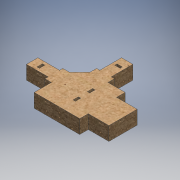
# Autodesk Inventor part: BearingStand
Saved by Autodesk Inventor 2016 (Build 200138000, 138)
## iProperties
Created: 2015-11-23
Part Number: BearingStand
Material: MDF Medium Density Fiberboard
Document SubType Name: Modeling
Designer: m2memari
Density: 0.8 g/cm^3
Appearance: Cardboard - Corrugated
BearingDiameter: 24.000 mm
WoodThickness: 6.390 mm
BearingWidth: 7.000 mm
BearingShaftDiameter: 8.000 mm
ZipTieWidth: 2.500 mm
ZipTieThickness: 1.100 mm
ZipTieClearance: 1.000 mm
ZipTieDistance: 10.000 mm
BearingShaftOffset: 1.574 mm
BearingHolderHeight: 23.674 mm
LatchHeight: 13.147 mm
BearingSiliconeWidth: 13.200 mm
Author: m2memari
Autodesk Inventor part; units mm, degrees
ref_plane "YZ Plane" through (0, 0, 0) normal (1, 0, 0) x (0, 1, 0)
ref_plane "XZ Plane" through (0, 0, 0) normal (0, 1, 0) x (-1, 0, 0)
ref_plane "XY Plane" through (0, 0, 0) normal (0, 0, 1) x (1, 0, 0)
sketch "Sketch1" plane through (0, 0, 0) normal (0, 0, 1) x (1, 0, 0)
  line L0 (-2.6473, 22.1) -> (2.6473, 22.1)
  line L1 (2.6473, 22.1) -> (2.6473, 12)
  line L2 (2.6473, 12) -> (4.1473, 12)
  line L3 (4.1473, 12) -> (4.1473, 9)
  line L4 (4.1473, 9) -> (12.1473, 9)
  line L5 (0, 22.1) -> (0, 0) construction
  line L6 (-2.6473, 22.1) -> (-2.6473, 12)
  line L7 (-2.6473, 12) -> (-4.1473, 12)
  line L8 (-1.25, 18.6) -> (1.25, 18.6)
  line L9 (1.25, 18.6) -> (1.25, 17.5)
  line L10 (1.25, 17.5) -> (-1.25, 17.5)
  line L11 (-1.25, 17.5) -> (-1.25, 18.6)
  line L12 (-5, -12.1473) -> (12.1473, -12.1473)
  line L13 (12.1473, 9) -> (12.1473, 5)
  line L14 (12.1473, 5) -> (21.7323, 5)
  line L15 (21.7323, -8.1473) -> (12.1473, -8.1473)
  line L16 (12.1473, -8.1473) -> (12.1473, -12.1473)
  line L17 (3.0473, 3) -> (4.1473, 3)
  line L18 (4.1473, 3) -> (4.1473, 0.5)
  line L19 (4.1473, 0.5) -> (3.0473, 0.5)
  line L20 (3.0473, 0.5) -> (3.0473, 3)
  line L21 (-4.1473, 12) -> (-19.8527, 12) construction
  line L22 (0, 0) -> (-12, 12) construction
  line L23 (-22.1, 2.6473) -> (-22.1, -2.6473)
  line L24 (-22.1, -2.6473) -> (-12, -2.6473)
  line L25 (-12, -2.6473) -> (-12, -4.1473)
  line L26 (-12, -4.1473) -> (-9, -4.1473)
  line L27 (-9, -4.1473) -> (-9, -12.1473)
  line L28 (-22.1, 2.6473) -> (-12, 2.6473)
  line L29 (-12, 2.6473) -> (-12, 4.1473)
  line L30 (-18.6, 1.25) -> (-18.6, -1.25)
  line L31 (-18.6, -1.25) -> (-17.5, -1.25)
  line L32 (-17.5, -1.25) -> (-17.5, 1.25)
  line L33 (-17.5, 1.25) -> (-18.6, 1.25)
  line L34 (-9, -12.1473) -> (-5, -12.1473)
  line L35 (-12, 12) -> (-12, -12.1473) construction
  line L36 (-4.1473, 12) -> (-4.1473, 9)
  line L37 (-9, 4.1473) -> (-12, 4.1473)
  line L38 (-4.1473, 9) -> (-9, 4.1473)
  line L39 (21.7323, 5) -> (21.7323, -8.1473)
  line L40 (21.7323, -1.5737) -> (3.3412, -1.5737) construction
  line L41 (3.0473, -6.1473) -> (4.1473, -6.1473)
  line L42 (4.1473, -6.1473) -> (4.1473, -3.6473)
  line L43 (4.1473, -3.6473) -> (3.0473, -3.6473)
  line L44 (3.0473, -3.6473) -> (3.0473, -6.1473)
  line L45 (-22.1, 0) -> (21.7323, 0) construction
  point P0 (0, 17.5)
  point P1 (3.0473, 1.75)
  point P2 (-17.5, 0)
  point P3 (4.1473, 1.75)
  point P4 (4.1473, 10.5)
  dimension "d4" = 1.5
  dimension "d5" = 3
  dimension "d26" = 10.1
  dimension "d27" = 5.2946
  dimension "d31" = 2.5
  dimension "d32" = 1.1
  dimension "d35" = 5.5
  dimension "d37" = 9.585
  dimension "d41" = 1.1
  dimension "d42" = 2.5
  dimension "d45" = 2
  dimension "d61" = 45
  dimension "d70" = 8
  dimension "d72" = 12
  dimension "BearingShaftOffset" = 1.5737
  dimension "BearingHolderHeight" = 23.6737
  dimension "LatchHeight" = 13.1473
  dimension "d95" = 24.1473
  constraints: 92 end point, 22 symmetric about line, 11 perpendicular, 7 midpoint, 6 horizontal, 5 parallel, 4 vertical, 3 vertical alignment, 2 collinear, 2 point on line
  measures "d4" distance of L1.end L2.end
  measures "d5" distance of L2.end L3.end
  measures "d26" distance of L0.end L1.end
  measures "d27" distance of L0.start L0.end
  measures "d31" distance of L8.start L8.end
  measures "d32" distance of L8.end L9.end
  measures "d35" distance between parallel lines of L7 L10
  measures "d37" distance of L13.end L14.end
  measures "d41" distance of L18.end L19.end
  measures "d42" distance of L17.end L18.end
  measures "d45" distance between parallel lines of L14 L17
  measures "d61" angle of L5 L22
  measures "d70" distance of L3.end L4.end
  measures "d72" distance between parallel lines of L35 L5
  measures "BearingShaftOffset" distance between parallel lines of L40 L45
  measures "BearingHolderHeight" distance between parallel lines of L40 L0
  measures "LatchHeight" distance between parallel lines of L15 L14
  measures "d95" distance between parallel lines of L35 L13
extrude "Extrusion2" add sketch "Sketch1" along normal blind 6.39
equation "\"BearingDiameter\" = 24"
equation "\"WoodThickness\" = 6.39"
equation "\"BearingWidth\" = 7"
equation "\"BearingShaftDiameter\" = 8"
equation "\"ZipTieWidth\" = 2.5"
equation "\"ZipTieThickness\" = 1.1"
equation "\"ZipTieClearance\" = 1"
equation "\"ZipTieDistance\" = 10"
equation "\"BearingSiliconeWidth\" = 13.2"
body "Solid2"
